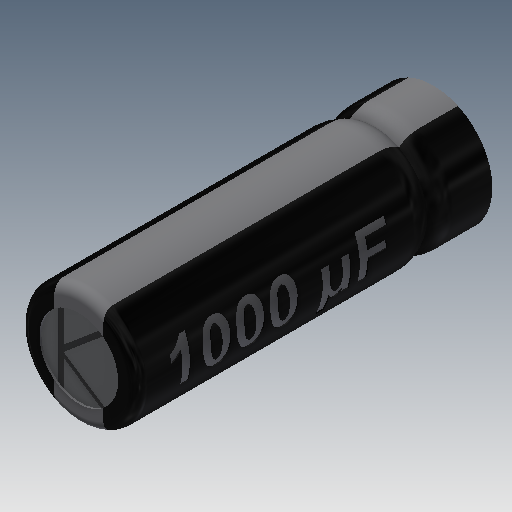
# Autodesk Inventor part: config - capasitor 1000 μF
Saved by Autodesk Inventor 2019.1 (Build 231200000, 200)
## iProperties
Company: Autodesk Asia Pte. Ltd.
Created: 2005-12-06
Part Number: config - capasitor 1000 μF
Document SubType Name: Modeling
Designer: Simon.Ng@autodesk.com
Stock Number: config - capasitor 1000 μF
Density: 1 g/cm^3
Material: Generic
Mass: 0.502546 g
Surface Area: 3.9754 cm^2
Volume: 0.502546 cm^3
Appearance: Glossy - Black
Title: PC Demo
Author: Simon.Ng@autodesk.com
Autodesk Inventor part; units mm, degrees
ref_plane "YZ Plane" through (0, 0, 0) normal (1, 0, 0) x (0, 1, 0)
ref_plane "XZ Plane" through (0, 0, 0) normal (0, 1, 0) x (-1, 0, 0)
ref_plane "XY Plane" through (0, 0, 0) normal (0, 0, 1) x (1, 0, 0)
sketch "Sketch1" plane through (0, 0, 0) normal (0, 0, 1) x (1, 0, 0)
  line L0 (0, 4.8) -> (0, -3.6) construction
  line L1 (-3.6, 0) -> (4.8, 0) construction
  circle A0 centre (0, 0) radius 3
  dimension "d0" = 6
  constraints: 2 point on line, 1 centre point
  measures "d0" diameter of A0
extrude "Extrusion1" add sketch "Sketch1" along normal blind 18
sketch "Sketch6" plane through (0, 0, 0) normal (1, 0, 0) x (0, 1, 0)
  line L0 (0, 29.25) -> (0, -2.25) projected
  line L1 (3, 0) -> (3, 18) projected
  line L2 (3, 4) -> (3, 2)
  line L3 (3, 3) -> (2.7, 3) construction
  line L4 (-3, 0) -> (3, 0) construction
  arc A0 (2.7, 3) -> (3, 4) centre (1.1833, 4) ccw
  arc A1 (3, 2) -> (2.7, 3) centre (1.1833, 2) ccw
  point P0 (0, 0)
  dimension "d16" = 2
  dimension "d17" = 3
  dimension "d18" = 0.3
  constraints: 4 end point, 4 point on circle, 2 centre point, 2 point on line, 2 tangent, 1 collinear, 1 horizontal, 1 midpoint
  measures "d16" distance of L2.start L2.end
  measures "d17" distance between parallel lines of L4 L3
  measures "d18" distance of L3.start L3.end
revolve "Revolution1" cut sketch "Sketch6" angle 360 about axis through (0, 0, 0) along (0, 0, -1)
sketch "Sketch2" plane through (0, 0, 18) normal (0, 0, 1) x (1, 0, 0)
  circle A0 centre (0, 0) radius 3 projected
  circle A1 centre (0, 0) radius 2
  dimension "d3" = 1
  constraints: 1 centre point, 1 coincident
  measures "d3" radial gap between concentric circles of A1 A0
extrude "Extrusion2" cut sketch "Sketch2" against normal blind 0.1 contours A1
sketch "Sketch3" plane through (0, 0, 17.9) normal (0, 0, 1) x (1, 0, 0)
  line L0 (-1.157, 1.8162) -> (-0.8695, 1.8162)
  line L1 (-0.8695, 1.8162) -> (-0.8695, -1.8349)
  line L2 (-0.8695, -1.8349) -> (-1.157, -1.8349)
  line L3 (-1.157, -1.8349) -> (-1.157, 1.8162)
  line L4 (-0.8695, -0.2083) -> (-1.0297, -0.0178)
  line L5 (-1.0297, -0.0178) -> (1.0822, 1.7578)
  line L6 (1.0822, 1.7578) -> (1.2424, 1.5673)
  line L7 (1.2424, 1.5673) -> (-0.8695, -0.2083)
  line L8 (-0.8695, -0.2083) -> (-0.9848, -0.3818)
  line L9 (-0.9848, -0.3818) -> (1.3396, -1.9264)
  line L10 (1.3396, -1.9264) -> (1.4549, -1.7529)
  line L11 (1.4549, -1.7529) -> (-0.8695, -0.2083)
  circle A0 centre (0, 0) radius 2 projected
  constraints: 24 end point, 6 parallel, 3 perpendicular, 1 horizontal, 1 point on line, 2 other
extrude "Extrusion3" cut sketch "Sketch3" against normal blind 0.05 contours L0 L1 A0 L3 | A0 L1 L5 L4 L8 L9 L3 | A0 L1 L2 L3 | L5 A0 L7 L1 | L1 L4 L5 | L5 L6 A0 | L11 A0 L9 L1 | L1 L9 L8 | A0 L11 L10 L9
fillet "Fillet1" radius 0.5 1 edges at (-3, 0, 18)
sketch "Sketch5" plane through (0, 0, 18) normal (0, 0, 1) x (1, 0, 0)
  circle A0 centre (0, 0) radius 2 projected
  circle A1 centre (0, 0) radius 3 projected
  line L0 (1.25, 1.5612) -> (1.25, -4)
  line L1 (1.25, -4) -> (-1.25, -4)
  line L2 (-1.25, -4) -> (-1.25, 1.5612)
  line L3 (0, -3.6) -> (0, 4.8) projected
  point P0 (0, -3)
  point P1 (0, -3)
  dimension "d12" = 1
  dimension "d13" = 2.5
  constraints: 6 end point, 2 point on circle, 1 coincident, 1 parallel, 1 point on line, 1 vertical alignment, 2 other
  measures "d12" distance from line of L1 point (0, -3)
  measures "d13" distance of L0.end L1.end
split_face "Split1"
ref_plane "Work Plane1" through (10, 0, 0) normal (1, 0, 0) x (0, 1, 0)
sketch "Sketch4" plane through (10, 0, 0) normal (1, 0, 0) x (0, 0, -1)
  line L0 (-16.5187, 1.3024) -> (-0.9104, 1.3024) construction
  line L1 (-0.9104, 1.3024) -> (-0.9104, -2.5368) construction
  line L2 (-0.9104, -2.5368) -> (-16.5187, -2.5368) construction
  line L3 (-16.5187, -2.5368) -> (-16.5187, 1.3024) construction
  line L4 (-15.308, -0.906) -> (-15.7305, -0.906)
  line L5 (-15.7305, -0.906) -> (-15.7305, 0.6819)
  spline S0 degree 2 poles (-15.7305, 0.6819) (-15.962, 0.4673) (-16.2755, 0.3633) knots 0 0 0 1 1 1
  line L6 (-16.2755, 0.3633) -> (-16.2755, 0.7457)
  spline S1 degree 3 poles (-16.2755, 0.7457) (-16.1095, 0.7993) (-15.7222, 1.1011) (-15.6501, 1.3024) knots 0 0 0 0 1 1 1 1
  line L7 (-15.6501, 1.3024) -> (-15.308, 1.3024)
  line L8 (-15.308, 1.3024) -> (-15.308, -0.906)
  spline S2 degree 2 poles (-13.9665, 1.3024) (-13.6462, 1.3024) (-13.4668, 1.0743) knots 0 0 0 1 1 1
  spline S3 degree 2 poles (-13.4668, 1.0743) (-13.2522, 0.8043) (-13.2522, 0.1789) knots 0 0 0 1 1 1
  spline S4 degree 2 poles (-13.2522, 0.1789) (-13.2522, -0.4449) (-13.4685, -0.7182) knots 0 0 0 1 1 1
  spline S5 degree 2 poles (-13.4685, -0.7182) (-13.6462, -0.9429) (-13.9665, -0.9429) knots 0 0 0 1 1 1
  spline S6 degree 3 poles (-13.9665, -0.9429) (-14.2885, -0.9429) (-14.6809, -0.4499) (-14.6809, 0.1839) knots 0 0 0 0 1 1 1 1
  spline S7 degree 2 poles (-14.6809, 0.1839) (-14.6809, 0.8043) (-14.4645, 1.0777) knots 0 0 0 1 1 1
  spline S8 degree 2 poles (-14.4645, 1.0777) (-14.2868, 1.3024) (-13.9665, 1.3024) knots 0 0 0 1 1 1
  spline S9 degree 3 poles (-13.9665, 0.9519) (-14.0437, 0.9519) (-14.1627, 0.8547) (-14.1962, 0.7289) knots 0 0 0 0 1 1 1 1
  spline S10 degree 2 poles (-14.1962, 0.7289) (-14.2398, 0.5662) (-14.2398, 0.1789) knots 0 0 0 1 1 1
  spline S11 degree 4 poles (-14.2398, 0.1789) (-14.2398, -0.2068) (-14.161, -0.4969) (-14.0437, -0.5925) (-13.9665, -0.5925) knots 0 0 0 0 0 1 1 1 1 1
  spline S12 degree 3 poles (-13.9665, -0.5925) (-13.8894, -0.5925) (-13.7703, -0.4952) (-13.7368, -0.3694) knots 0 0 0 0 1 1 1 1
  spline S13 degree 2 poles (-13.7368, -0.3694) (-13.6932, -0.2068) (-13.6932, 0.1789) knots 0 0 0 1 1 1
  spline S14 degree 4 poles (-13.6932, 0.1789) (-13.6932, 0.5662) (-13.772, 0.8547) (-13.8894, 0.9519) (-13.9665, 0.9519) knots 0 0 0 0 0 1 1 1 1 1
  spline S15 degree 2 poles (-12.2578, 1.3024) (-11.9376, 1.3024) (-11.7581, 1.0743) knots 0 0 0 1 1 1
  spline S16 degree 2 poles (-11.7581, 1.0743) (-11.5435, 0.8043) (-11.5435, 0.1789) knots 0 0 0 1 1 1
  spline S17 degree 2 poles (-11.5435, 0.1789) (-11.5435, -0.4449) (-11.7598, -0.7182) knots 0 0 0 1 1 1
  spline S18 degree 2 poles (-11.7598, -0.7182) (-11.9376, -0.9429) (-12.2578, -0.9429) knots 0 0 0 1 1 1
  spline S19 degree 3 poles (-12.2578, -0.9429) (-12.5798, -0.9429) (-12.9722, -0.4499) (-12.9722, 0.1839) knots 0 0 0 0 1 1 1 1
  spline S20 degree 2 poles (-12.9722, 0.1839) (-12.9722, 0.8043) (-12.7559, 1.0777) knots 0 0 0 1 1 1
  spline S21 degree 2 poles (-12.7559, 1.0777) (-12.5781, 1.3024) (-12.2578, 1.3024) knots 0 0 0 1 1 1
  spline S22 degree 3 poles (-12.2578, 0.9519) (-12.335, 0.9519) (-12.454, 0.8547) (-12.4876, 0.7289) knots 0 0 0 0 1 1 1 1
  spline S23 degree 2 poles (-12.4876, 0.7289) (-12.5312, 0.5662) (-12.5312, 0.1789) knots 0 0 0 1 1 1
  spline S24 degree 4 poles (-12.5312, 0.1789) (-12.5312, -0.2068) (-12.4523, -0.4969) (-12.335, -0.5925) (-12.2578, -0.5925) knots 0 0 0 0 0 1 1 1 1 1
  spline S25 degree 3 poles (-12.2578, -0.5925) (-12.1807, -0.5925) (-12.0616, -0.4952) (-12.0281, -0.3694) knots 0 0 0 0 1 1 1 1
  spline S26 degree 2 poles (-12.0281, -0.3694) (-11.9845, -0.2068) (-11.9845, 0.1789) knots 0 0 0 1 1 1
  spline S27 degree 4 poles (-11.9845, 0.1789) (-11.9845, 0.5662) (-12.0633, 0.8547) (-12.1807, 0.9519) (-12.2578, 0.9519) knots 0 0 0 0 0 1 1 1 1 1
  spline S28 degree 2 poles (-10.5491, 1.3024) (-10.2289, 1.3024) (-10.0495, 1.0743) knots 0 0 0 1 1 1
  spline S29 degree 2 poles (-10.0495, 1.0743) (-9.8348, 0.8043) (-9.8348, 0.1789) knots 0 0 0 1 1 1
  spline S30 degree 2 poles (-9.8348, 0.1789) (-9.8348, -0.4449) (-10.0511, -0.7182) knots 0 0 0 1 1 1
  spline S31 degree 2 poles (-10.0511, -0.7182) (-10.2289, -0.9429) (-10.5491, -0.9429) knots 0 0 0 1 1 1
  spline S32 degree 3 poles (-10.5491, -0.9429) (-10.8711, -0.9429) (-11.2635, -0.4499) (-11.2635, 0.1839) knots 0 0 0 0 1 1 1 1
  spline S33 degree 2 poles (-11.2635, 0.1839) (-11.2635, 0.8043) (-11.0472, 1.0777) knots 0 0 0 1 1 1
  spline S34 degree 2 poles (-11.0472, 1.0777) (-10.8694, 1.3024) (-10.5491, 1.3024) knots 0 0 0 1 1 1
  spline S35 degree 3 poles (-10.5491, 0.9519) (-10.6263, 0.9519) (-10.7453, 0.8547) (-10.7789, 0.7289) knots 0 0 0 0 1 1 1 1
  spline S36 degree 2 poles (-10.7789, 0.7289) (-10.8225, 0.5662) (-10.8225, 0.1789) knots 0 0 0 1 1 1
  spline S37 degree 4 poles (-10.8225, 0.1789) (-10.8225, -0.2068) (-10.7437, -0.4969) (-10.6263, -0.5925) (-10.5491, -0.5925) knots 0 0 0 0 0 1 1 1 1 1
  spline S38 degree 3 poles (-10.5491, -0.5925) (-10.472, -0.5925) (-10.353, -0.4952) (-10.3194, -0.3694) knots 0 0 0 0 1 1 1 1
  spline S39 degree 2 poles (-10.3194, -0.3694) (-10.2758, -0.2068) (-10.2758, 0.1789) knots 0 0 0 1 1 1
  spline S40 degree 4 poles (-10.2758, 0.1789) (-10.2758, 0.5662) (-10.3546, 0.8547) (-10.472, 0.9519) (-10.5491, 0.9519) knots 0 0 0 0 0 1 1 1 1 1
  line L9 (-8.6141, 0.6886) -> (-8.1915, 0.6886)
  line L10 (-8.1915, 0.6886) -> (-8.1915, -0.0357)
  spline S41 degree 4 poles (-8.1915, -0.0357) (-8.1915, -0.2386) (-8.1496, -0.4667) (-8.002, -0.6075) (-7.8981, -0.6075) knots 0 0 0 0 0 1 1 1 1 1
  spline S42 degree 4 poles (-7.8981, -0.6075) (-7.7908, -0.6075) (-7.6348, -0.46) (-7.5895, -0.2504) (-7.5895, -0.0408) knots 0 0 0 0 0 1 1 1 1 1
  line L11 (-7.5895, -0.0408) -> (-7.5895, 0.6886)
  line L12 (-7.5895, 0.6886) -> (-7.167, 0.6886)
  line L13 (-7.167, 0.6886) -> (-7.167, -0.906)
  line L14 (-7.167, -0.906) -> (-7.556, -0.906)
  line L15 (-7.556, -0.906) -> (-7.556, -0.7132)
  spline S43 degree 2 poles (-7.556, -0.7132) (-7.6734, -0.9412) (-7.8763, -0.9412) knots 0 0 0 1 1 1
  spline S44 degree 2 poles (-7.8763, -0.9412) (-8.0909, -0.9412) (-8.1915, -0.7132) knots 0 0 0 1 1 1
  line L16 (-8.1915, -0.7132) -> (-8.1915, -1.513)
  line L17 (-8.1915, -1.513) -> (-8.6141, -1.513)
  line L18 (-8.6141, -1.513) -> (-8.6141, 0.6886)
  line L19 (-6.726, -0.906) -> (-6.726, 1.294)
  line L20 (-6.726, 1.294) -> (-5.2152, 1.294)
  line L21 (-5.2152, 1.294) -> (-5.2152, 0.9217)
  line L22 (-5.2152, 0.9217) -> (-6.2816, 0.9217)
  line L23 (-6.2816, 0.9217) -> (-6.2816, 0.4019)
  line L24 (-6.2816, 0.4019) -> (-5.361, 0.4019)
  line L25 (-5.361, 0.4019) -> (-5.361, 0.0297)
  line L26 (-5.361, 0.0297) -> (-6.2816, 0.0297)
  line L27 (-6.2816, 0.0297) -> (-6.2816, -0.906)
  line L28 (-6.2816, -0.906) -> (-6.726, -0.906)
  constraints: 2 other
emboss "Emboss1" sketch "Sketch4" operation cut depth 0.05 direction (1, 0, 0) wrap yes faces at (-0.3679, 2.9774, 8.5) (-0.3679, 2.9774, 8.5) (-0.3679, 2.9774, 8.5) (-0.3679, 2.9774, 1.3333) (-0.3679, 2.9774, 1.3333) (-0.3679, 2.9774, 1.3333) (-0.3679, 2.9774, 1.3333) (-0.3679, 2.9774, 8.5)
body "Solid1"
